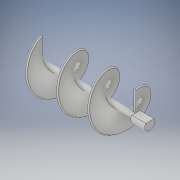
# Autodesk Inventor part: Шнек
Saved by Autodesk Inventor 2019 (Build 230136000, 136)
## iProperties
Created: 2019-04-26
Part Number: Шнек
Material: Типовые
Document SubType Name: Modeling
Designer: BarmanKaktus
Density: 1 g/cm^3
Appearance: По умолчанию
Author: BarmanKaktus
Autodesk Inventor part; units mm, degrees
ref_plane "YZ Plane" through (0, 0, 0) normal (1, 0, 0) x (0, 1, 0)
sketch "Эскиз1" plane through (0, 0, 0) normal (0, 0, 1) x (1, 0, 0)
  line L0 (0, 0) -> (-2, 0)
  line L1 (-2, 0) -> (-2, 19)
  line L2 (-1, 20) -> (-1, 20)
  line L3 (0, 19) -> (0, 0)
  arc A0 (-1, 20) -> (-2, 19) centre (-1, 19) ccw
  arc A1 (0, 19) -> (-1, 20) centre (-1, 19) ccw
  line L4 (-3.2847, -2.5) -> (39.0714, -2.5)
  point P0 (-2, 20)
  point P1 (0, 20)
  dimension "d0" = 2
  dimension "d1" = 20
  dimension "d2" = 1
  dimension "d3" = 2.5
  constraints: 10 end point, 4 point on circle, 4 point on line, 4 tangent, 2 centre point, 2 horizontal, 2 parallel, 1 concentric, 1 perpendicular
  measures "d0" distance of point (-2, 20) point (0, 20)
  measures "d1" distance of L0.end point (-2, 20)
  measures "d2" radius of A0
  measures "d3" distance between parallel lines of L0 L4
coil "Пружина1" sketch "Эскиз1" operation add axis through (-3.2847, -2.5, 0) along (1, 0, 0) pitch 30 turns 3 hand right
ref_plane "РабПлоскость1" through (90, 19, 0) normal (1, 0, 0) x (0, 1, 0)
sketch "Эскиз2" plane through (90, 19, 0) normal (1, 0, 0) x (0, 1, 0)
  circle A0 centre (-21.5, 0) radius 2.5
  point P0 (-19, 0)
  dimension "d13" = 5
  dimension "d14" = 2.5
  constraints: 1 centre point
  measures "d13" diameter of A0
  measures "d14" distance of point (-19, 0) A0.centre
extrude "Выдавливание1" add sketch "Эскиз2" against normal blind 92
sketch "Эскиз3" plane through (-2, -2.5, 0) normal (-1, 0, 0) x (0, 0, 1)
  line L0 (0, 2.5) -> (-2.5, 0)
  circle A0 centre (0, 0) radius 2.5 projected
  line L1 (0, -2.5) -> (2.5, 0)
  line L2 (0, 2.5) -> (0, 21.5) projected
  line L3 (0, 2.5) -> (2.5, 0)
  line L4 (0, -2.5) -> (-2.5, 0)
  constraints: 8 end point, 3 point on circle, 2 parallel, 1 perpendicular
extrude "Выдавливание2" add sketch "Эскиз3" along normal blind 8 contours L3 L1 L4 L0
sketch "Эскиз4" plane through (-10, -2.5, 0) normal (-1, 0, 0) x (0, 0, 1)
  circle A0 centre (0, 0) radius 1.7678
  point P0 (0, 2.5)
  constraints: 1 centre point
extrude "Выдавливание3" add sketch "Эскиз4" along normal blind 2
sketch "Эскиз5" plane through (90, -2.5, 0) normal (1, 0, 0) x (0, 0, -1)
  point P0 (0, 2.5)
ref_plane "РабПлоскость2" through (90, -2.5, 0) normal (1, 0, 0) x (0, 0, -1)
sketch "Эскиз6" plane through (90, -2.5, 0) normal (1, 0, 0) x (0, 0, -1)
  circle A0 centre (0, 0) radius 5
  line L0 (0, 3) -> (4, 3)
  line L1 (-4, 3) -> (0, 3)
  point P0 (0, 2.5)
  dimension "d22" = 10
  dimension "d24" = 3
  constraints: 4 end point, 2 collinear, 2 point on circle, 1 centre point, 1 point on line
  measures "d22" diameter of A0
  measures "d24" distance of L0.start A0.centre
extrude "Выдавливание4" add sketch "Эскиз6" along normal blind 13.5 contours A0 L1 L0 picked at (0.1095, -2.3082)
